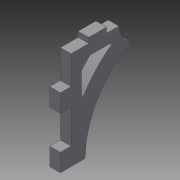
# Autodesk Inventor part: Harness Pusher 2
Saved by Autodesk Inventor 2015 (Build 190159000, 159)
## iProperties
Created: 2014-07-21
Part Number: Harness Pusher 2
Material: Generic
Document SubType Name: Modeling
Designer: STACKPOLE
Density: 1 g/cm^3
Appearance: Default
Author: STACKPOLE
Autodesk Inventor part; units mm, degrees
ref_plane "YZ Plane" through (0, 0, 0) normal (1, 0, 0) x (0, 1, 0)
ref_plane "XZ Plane" through (0, 0, 0) normal (0, 1, 0) x (-1, 0, 0)
ref_plane "XY Plane" through (0, 0, 0) normal (0, 0, 1) x (1, 0, 0)
sketch "Sketch1" plane through (0, 0, 0) normal (1, 0, 0) x (0, 1, 0)
  circle A0 centre (-8.4812, -1.44) radius 50 construction
  line L0 (-46.4812, 56.56) -> (-56.4812, 56.56)
  line L1 (-56.4812, 56.56) -> (-56.4812, 53.56)
  line L2 (-66.4812, 27.56) -> (-72.4812, 27.56)
  line L3 (-72.4812, 27.56) -> (-72.4812, 37.56)
  line L4 (-72.4812, 37.56) -> (-66.4812, 37.56)
  arc A1 (-44.3506, 33.3937) -> (-32.2509, 42.5487) centre (-8.4812, -1.44) ccw construction
  line L5 (-66.4812, 53.56) -> (-66.4812, 37.56)
  line L6 (-56.4812, 53.56) -> (-66.4812, 53.56)
  line L7 (-66.4812, 53.56) -> (-45.3047, 32.3835) construction
  line L8 (-58.4812, -1.44) -> (-65.4812, -1.44)
  line L9 (-65.4812, -1.44) -> (-72.4812, -1.44)
  line L10 (-72.4812, -1.44) -> (-72.4812, 8.56)
  line L11 (-72.4812, 8.56) -> (-66.4812, 8.56)
  line L12 (-66.4812, 27.56) -> (-66.4812, 8.56)
  arc A2 (-32.2509, 42.5487) -> (-58.4812, -1.44) centre (-8.4812, -1.44) ccw
  arc A3 (-39.4812, 53.56) -> (-32.2509, 42.5487) centre (-27.4812, 53.56) ccw
  line L13 (-46.4812, 56.56) -> (-46.4812, 53.56)
  line L14 (-46.4812, 53.56) -> (-39.4812, 53.56)
  line L15 (-48.4406, 53.56) -> (-18.7746, 53.56) construction
  point P0 (-30.5194, 43.4412)
  dimension "d6" = 50
  dimension "d8" = 10
  dimension "d10" = 3
  dimension "d11" = 10
  dimension "d12" = 6
  dimension "d18" = 10
  dimension "d23" = 45
  dimension "d30" = 10
  dimension "d31" = 6
  dimension "d32" = 19
  dimension "d38" = 58
  dimension "d50" = 7
  dimension "d51" = 16
  dimension "d57" = 12
  dimension "d69" = 7
  dimension "d70" = 7
  constraints: 32 end point, 13 point on circle, 5 horizontal, 4 centre point, 3 parallel, 3 perpendicular, 3 vertical, 2 point on line, 1 coincident, 1 horizontal alignment, 1 vertical alignment
  measures "d6" radius of A0
  measures "d8" distance of L0.start L0.end
  measures "d10" distance of L0.end L1.end
  measures "d11" distance of L2.end L3.end
  measures "d12" distance of L2.start L2.end
  measures "d18" distance of L1.end L5.start
  measures "d23" angle of L6 L7
  measures "d30" distance of L9.end L10.end
  measures "d31" distance of L11.end L10.end
  measures "d32" distance of L2.start L11.end
  measures "d38" distance from line of L12 A0.centre
  measures "d50" distance of L8.start L8.end
  measures "d51" distance between parallel lines of L6 L4
  measures "d57" radius of A3
  measures "d69" distance of L8.end L9.end
  measures "d70" distance of L13.end L14.end
extrude "Extrusion2" add sketch "Sketch1" along normal blind 6
fillet "Fillet3" radius 0.75 2 edges at (3, -32.2509, 42.5487) (3, -58.4812, -1.44)
sketch "Sketch2" plane through (6, 0, 0) normal (1, 0, 0) x (0, 0, -1)
  line L0 (-27.7662, -60.4812) -> (-47.56, -60.4812)
  line L1 (-47.56, -60.4812) -> (-47.56, -42.4812)
  line L2 (-53.56, -56.4812) -> (-53.56, -66.4812) projected
  line L3 (-53.56, -66.4812) -> (-37.56, -66.4812) projected
  line L4 (-56.56, -46.4812) -> (-56.56, -56.4812) projected
  arc A0 (-41.8649, -33.4749) -> (0.701, -58.4757) centre (1.44, -8.4812) ccw projected
  arc A1 (-47.56, -42.4812) -> (-27.7662, -60.4812) centre (1.44, -8.4812) ccw
  point P0 (-53.56, -39.4812)
  dimension "d42" = 6
  dimension "d43" = 6
  dimension "d73" = 3
  constraints: 4 end point, 2 parallel, 2 point on circle, 1 centre point, 1 concentric, 1 horizontal, 1 perpendicular
  measures "d42" distance between parallel lines of L3 L0
  measures "d43" distance between parallel lines of L2 L1
  measures "d73" vertical distance of L1.end point (-53.56, -39.481)
extrude "Extrusion5" cut sketch "Sketch2" against normal blind 10
fillet "Fillet7" radius 0.5 3 edges at (3, -42.4812, 47.56) (3, -60.4812, 47.56) (3, -60.4812, 27.7662)
body "Solid2"
